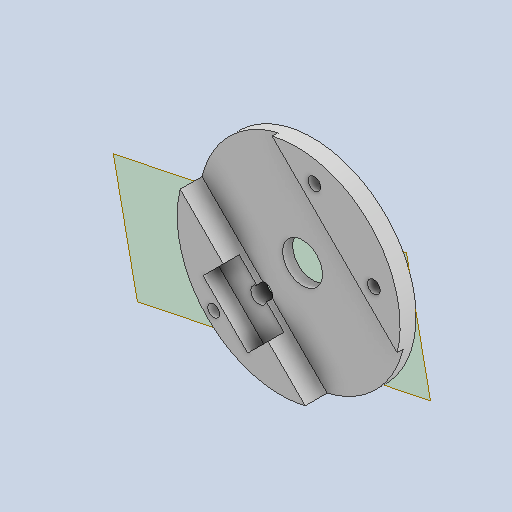
# Autodesk Inventor part: Matchboxscope_sample_v0
Saved by Autodesk Inventor 2022 (Build 260153000, 153)
## iProperties
Created: 2022-03-21
Part Number: Matchboxscope_sample_v0
Material: Generic
Document SubType Name: Modeling
Designer: Prakash Lab
Density: 1 g/cm^3
Appearance: Default
Author: Prakash Lab
Autodesk Inventor part; units mm, degrees
ref_plane "YZ Plane" through (0, 0, 0) normal (1, 0, 0) x (0, 1, 0)
ref_plane "XZ Plane" through (0, 0, 0) normal (0, 1, 0) x (-1, 0, 0)
ref_plane "XY Plane" through (0, 0, 0) normal (0, 0, 1) x (1, 0, 0)
ref_plane "Work Plane1" through (20.4075, 0, 0) normal (0, 0, -1) x (-0.9792327, -0.2027397, 0)
sketch "Sketch1" plane through (0, 0, 0) normal (0, 0, 1) x (0.9792327, -0.2027397, 0)
  circle A0 centre (8.0687, 11.3576) radius 25.9979 projected
  circle A1 centre (8.0703, 11.3562) radius 3.8103 projected
  circle A2 centre (8.0703, 11.3562) radius 5
  point P0 (0, 0)
  dimension "d0" = 10
  constraints: 1 centre point, 1 coincident
  measures "d0" diameter of A2
extrude "Extrusion1" add sketch "Sketch1" along normal blind 4 contours A0
sketch "Sketch2" plane through (10.2037, 9.4859, 4) normal (0, 0, 1) x (1, 0, 0)
  line L0 (-10.2037, 54.0449) -> (-10.2037, -50.593) projected
  line L1 (-54.0467, -9.4859) -> (50.5907, -9.4859) projected
  line L2 (-15.9479, -15.1669) -> (4.4725, 20.2023)
  line L3 (4.4725, 20.2023) -> (19.4213, 5.2535)
  line L4 (19.4213, 5.2535) -> (-15.9479, -15.1669)
  line L5 (-39.0985, 39.0967) -> (35.6425, -35.6447)
  line L6 (-0.781, 0) -> (9.2905, 10.0715)
  line L7 (-0.781, 0) -> (13.4622, 0) construction
  line L8 (-15.9479, -15.1669) -> (-0.781, 0)
  circle A0 centre (4.4725, 20.2023) radius 1.6
  circle A1 centre (19.4213, 5.2535) radius 1.6
  circle A2 centre (-15.9479, -15.1669) radius 1.6 construction
  circle A3 centre (-16.8292, -16.048) radius 1.5
  dimension "d17" = 18
  dimension "d18" = 22
  dimension "d19" = 30
  dimension "d20" = 45
  dimension "d21" = 15
  dimension "d22" = 3.2
  dimension "d23" = 3.2
  dimension "d24" = 3.2
  dimension "d39" = 3
  constraints: 14 end point, 4 centre point, 3 coincident, 1 collinear, 1 equal length, 1 horizontal, 1 parallel, 3 other
  measures "d17" distance from line of L6.start L3
  measures "d18" distance from line of L5 L2.start
  measures "d19" angle of L2 L4
  measures "d20" angle of L7 L6
  measures "d21" angle of L2 L6
  measures "d22" diameter of A0
  measures "d23" diameter of A1
  measures "d24" diameter of A2
  measures "d39" diameter of A3
extrude "Extrusion2" cut sketch "Sketch2" against normal through all contours A0 L3 L2 | L2 L3 A0 | A3 L8 L2 | L2 L4 A3 | A3 L4 L8 | A1 L4 L3 | L3 L4 A1
sketch "Sketch3" plane through (10.2037, 9.4859, 4) normal (0, 0, 1) x (1, 0, 0)
  line L0 (-35.7047, 22.4019) -> (13.1872, -35.1292) projected
  line L1 (32.542, -18.6808) -> (-16.3499, 38.8503) projected
  line L2 (40.2702, -21.1784) -> (-21.1782, 40.2703)
  line L3 (-21.1782, 40.2703) -> (-40.2702, 21.1784)
  line L4 (-40.2702, 21.1784) -> (21.1782, -40.2703)
  line L5 (21.1782, -40.2703) -> (40.2702, -21.1784)
  line L6 (40.2702, -21.1784) -> (-40.2702, 21.1784) construction
  line L7 (-21.1782, 40.2703) -> (21.1782, -40.2703) construction
  point P0 (0, 0)
  dimension "d16" = 27
  constraints: 12 end point, 2 midpoint, 2 parallel, 1 perpendicular
  measures "d16" distance of L3.end L2.end
extrude "Extrusion3" cut sketch "Sketch3" against normal blind 1.5
sketch "Sketch4" plane through (0, 0, 4) normal (0, 0, 1) x (0.9792327, -0.2027397, 0)
  circle A0 centre (0.9966, -1.342) radius 2 projected
extrude "Extrusion4" cut sketch "Sketch4" against normal blind 25.4
sketch "Sketch6" plane through (0, 0, 4) normal (0, 0, 1) x (0.9792327, -0.2027397, 0)
  line L0 (-8.7836, -2.1144) -> (-5.1612, 3.3996) projected
  line L1 (4.1709, -10.6249) -> (-8.7836, -2.1144) projected
  line L2 (4.1709, -10.6249) -> (7.7934, -5.1109) projected
  circle A0 centre (-5.1575, -7.7691) radius 1.5 projected
  arc A1 (0.095, 0.4433) -> (2.9931, -1.4605) centre (0.9966, -1.342) ccw projected
  line L3 (0.095, 0.4433) -> (-17.9131, 12.2738) projected
  arc A2 (-17.9131, 12.2738) -> (19.2256, -12.1245) centre (8.0687, 11.3576) ccw projected
  line L4 (19.2256, -12.1245) -> (2.9931, -1.4605) projected
  line L5 (-8.7836, -2.1144) -> (4.1709, -10.6249)
  line L6 (4.1709, -10.6249) -> (8.0213, -4.7639)
  line L7 (8.0213, -4.7639) -> (-4.9332, 3.7466)
  line L8 (-4.9332, 3.7466) -> (-8.7836, -2.1144)
  line L9 (-9.0606, -2.1717) -> (4.2283, -10.9019)
  line L10 (4.2283, -10.9019) -> (8.1885, -4.8737)
  line L11 (8.2983, -4.7065) -> (-4.9906, 4.0236)
  line L12 (-4.9906, 4.0236) -> (-5.1004, 3.8565)
  line L13 (-5.1004, 3.8565) -> (-9.0606, -2.1717)
  line L14 (8.1885, -4.8737) -> (8.2983, -4.7065)
  point P0 (0, 0)
  dimension "d44" = 0.2
  constraints: 20 end point, 7 parallel, 3 perpendicular, 2 point on line
  measures "d44" distance between parallel lines of L8 L12
extrude "Extrusion6" add sketch "Sketch6" along normal blind 4 contours L13 L9 L10 L4 A2 L3
body "Solid1"
